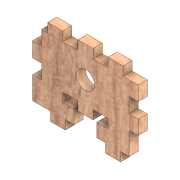
# Autodesk Inventor part: jotstick behuizing zijkant 2.1
Saved by Autodesk Inventor 2020.3 (Build 243373000, 373)
## iProperties
Created: 2020-12-09
Part Number: jotstick behuizing zijkant 2.1
Material: Wood (Birch)
Document SubType Name: Sheet Metal
Designer: Svend
Density: 0.55 g/cm^3
Sheet Metal Rule: Default_mm
Appearance: Birch - Natural Polished
Author: Svend
Autodesk Inventor part; units mm, degrees
ref_plane "YZ Plane" through (0, 0, 0) normal (1, 0, 0) x (0, 1, 0)
ref_plane "XZ Plane" through (0, 0, 0) normal (0, 1, 0) x (-1, 0, 0)
ref_plane "XY Plane" through (0, 0, 0) normal (0, 0, 1) x (1, 0, 0)
ref_plane "Work Plane1" through (20, 0, 0) normal (0, 0, 1) x (1, 0, 0)
sketch "Sketch1" plane through (20, 0, 0) normal (0, 0, 1) x (1, 0, 0)
  line L0 (-20, 0) -> (-10, 0)
  line L1 (-10, 0) -> (-10, 6)
  line L2 (-20, 6) -> (-10, 6)
  line L3 (-20, 0) -> (-20, 6)
  line L4 (0, 0) -> (10, 0)
  line L5 (10, 0) -> (10, 6)
  line L6 (0, 6) -> (10, 6)
  line L7 (0, 0) -> (0, 6)
  line L8 (20, 0) -> (30, 0)
  line L9 (30, 0) -> (30, 6)
  line L10 (20, 6) -> (30, 6)
  line L11 (20, 0) -> (20, 6)
  line L12 (-30, 0) -> (-24, 0)
  line L13 (-24, 0) -> (-24, 6)
  line L14 (-30, 6) -> (-24, 6)
  line L15 (-30, 0) -> (-30, 6)
  line L16 (-30, 0) -> (-20, 0)
  line L17 (-10, 0) -> (0, 0)
  line L18 (10, 0) -> (20, 0)
  line L19 (30, 0) -> (40, 0)
  line L20 (40, 0) -> (-24, 0)
  line L21 (-24, 0) -> (-24, -29)
  line L22 (-24, -29) -> (40, -29)
  line L23 (40, -29) -> (40, 0)
  line L24 (-24, -9.5) -> (-30, -9.5)
  line L25 (-30, -9.5) -> (-30, -19.5)
  line L26 (-30, -19.5) -> (-24, -19.5)
  line L27 (-24, -19.5) -> (-24, -9.5)
  line L28 (40, -19.5) -> (34, -19.5)
  line L29 (34, -19.5) -> (34, -9.5)
  line L30 (34, -9.5) -> (40, -9.5)
  line L31 (40, -9.5) -> (40, -19.5)
  line L32 (-24, -14.5) -> (40, -14.5) construction
  line L33 (-20, -29) -> (-10, -29)
  line L34 (-10, -29) -> (-10, -35)
  line L35 (-20, -35) -> (-10, -35)
  line L36 (-20, -29) -> (-20, -35)
  line L37 (0, -29) -> (10, -29)
  line L38 (10, -29) -> (10, -35)
  line L39 (0, -35) -> (10, -35)
  line L40 (0, -29) -> (0, -35)
  line L41 (20, -29) -> (30, -29)
  line L42 (30, -29) -> (30, -35)
  line L43 (20, -35) -> (30, -35)
  line L44 (20, -29) -> (20, -35)
  line L45 (-10, -29) -> (0, -29)
  line L46 (10, -29) -> (20, -29)
  point P0 (-30, -14.5)
  point P1 (34, -14.5)
  dimension "d0" = 29
  dimension "d1" = 6
  dimension "d2" = 10
  measures "d0" distance of L21.end L20.end
  measures "d1" distance of L26.end L25.end
  measures "d2" distance of L25.end L24.end
extrude "Plate1" add sketch "Sketch1" along normal blind 6 contours L3 L2 L1 L0 | L0 L17 L4 L18 L8 L19 L23 L30 L29 L28 L22 L21 L16 | L7 L6 L5 L4 | L21 L26 L25 L24 | L11 L10 L9 L8 | L22 L34 L35 L36 | L22 L38 L39 L40 | L22 L42 L43 L44
sketch "Sketch2" plane through (20, 0, 6) normal (0, 0, 1) x (1, 0, 0)
  line L0 (-24, -44) -> (-24, -29)
  line L1 (-18.25, -44) -> (-30, -44)
  line L2 (-2.5, -44) -> (-8.25, -44)
  line L3 (-2.5, -35.5) -> (-2.5, -44)
  line L4 (12, -35) -> (-2, -35)
  line L5 (10, -35) -> (0, -35) construction
  line L6 (5, -35) -> (5, 6) construction
  line L7 (0, 6) -> (10, 6) construction
  line L8 (40, -19.5) -> (34, -19.5)
  line L9 (34, -19.5) -> (34, -9.5)
  line L10 (34, -9.5) -> (40, -9.5)
  line L11 (40, 0) -> (40, -9.5)
  line L12 (30, 0) -> (40, 0)
  line L13 (30, 6) -> (30, 0)
  line L14 (20, 6) -> (30, 6)
  line L15 (20, 0) -> (20, 6)
  line L16 (10, 0) -> (20, 0)
  line L17 (10, 6) -> (10, 0)
  line L18 (0, 6) -> (10, 6)
  line L19 (0, 0) -> (0, 6)
  line L20 (-10, 0) -> (0, 0)
  line L21 (-10, 6) -> (-10, 0)
  line L22 (-20, 6) -> (-10, 6)
  line L23 (-20, 0) -> (-20, 6)
  line L24 (-24, 0) -> (-20, 0)
  line L25 (-24, -9.5) -> (-24, 0)
  line L26 (-30, -9.5) -> (-24, -9.5)
  line L27 (-30, -19.5) -> (-30, -9.5)
  line L28 (-24, -19.5) -> (-30, -19.5)
  line L29 (-24, -29) -> (-24, -19.5)
  line L30 (-20, -29) -> (-24, -29)
  line L31 (-20, -35) -> (-20, -29)
  line L32 (-10, -35) -> (-20, -35)
  line L33 (-10, -29) -> (-10, -35)
  line L34 (0, -29) -> (-10, -29)
  line L35 (0, -35) -> (0, -29)
  line L36 (10, -35) -> (0, -35)
  line L37 (10, -29) -> (10, -35)
  line L38 (20, -29) -> (10, -29)
  line L39 (20, -35) -> (20, -29)
  line L40 (30, -35) -> (20, -35)
  line L41 (30, -29) -> (30, -35)
  line L42 (40, -29) -> (30, -29)
  line L43 (40, -19.5) -> (40, -29)
  line L44 (-2.5, -44) -> (-2.5, -35)
  line L45 (-2.5, -35) -> (0, -35)
  line L46 (-8.25, -50) -> (-18.25, -50)
  line L47 (-18.25, -50) -> (-18.25, -44)
  line L48 (34, -44) -> (34, -29)
  line L49 (12.5, -44) -> (18.25, -44)
  line L50 (12.5, -35.5) -> (12.5, -44)
  line L51 (30, -29) -> (34, -29)
  line L52 (30, -35) -> (30, -29)
  line L53 (20, -35) -> (30, -35)
  line L54 (20, -29) -> (20, -35)
  line L55 (10, -29) -> (20, -29)
  line L56 (10, -35) -> (10, -29)
  line L57 (12.5, -44) -> (12.5, -35)
  line L58 (12.5, -35) -> (10, -35)
  line L59 (18.25, -50) -> (28.25, -50)
  line L60 (28.25, -50) -> (28.25, -44)
  line L61 (28.25, -44) -> (34, -44)
  line L62 (-24, -29) -> (-20, -29)
  line L63 (-20, -35) -> (-20, -29)
  line L64 (-20, -35) -> (-20, -29)
  line L65 (-20, -35) -> (-10, -35)
  line L66 (-10, -35) -> (-10, -29)
  line L67 (0, -29) -> (-10, -29)
  line L68 (0, -29) -> (0, -35)
  line L69 (-8.25, -44) -> (-8.25, -50)
  line L70 (18.25, -50) -> (18.25, -44)
  line L71 (34, -44) -> (34, -29)
  line L72 (28.25, -44) -> (40, -44)
  line L73 (12.5, -44) -> (18.25, -44)
  line L74 (12.5, -35.5) -> (12.5, -44)
  line L75 (30, -29) -> (34, -29)
  line L76 (30, -35) -> (30, -29)
  line L77 (20, -35) -> (30, -35)
  line L78 (20, -29) -> (20, -35)
  line L79 (10, -29) -> (20, -29)
  line L80 (10, -35) -> (10, -29)
  line L81 (12.5, -44) -> (12.5, -35)
  line L82 (12.5, -35) -> (10, -35)
  line L83 (18.25, -50) -> (28.25, -50)
  line L84 (28.25, -50) -> (28.25, -44)
  line L85 (34, -29) -> (30, -29)
  line L86 (30, -35) -> (30, -29)
  line L87 (30, -35) -> (30, -29)
  line L88 (30, -35) -> (20, -35)
  line L89 (20, -35) -> (20, -29)
  line L90 (10, -29) -> (20, -29)
  line L91 (10, -29) -> (10, -35)
  line L92 (18.25, -44) -> (18.25, -50)
  line L93 (-24, -44) -> (-30, -44)
  line L94 (-30, -44) -> (-30, -29)
  line L95 (-30, -29) -> (-24, -29)
  line L96 (-24, -29) -> (-24, -44)
  line L97 (-10, -29) -> (0, -29)
  line L98 (0, -29) -> (0, -35)
  line L99 (0, -35) -> (-10, -35)
  line L100 (-10, -35) -> (-10, -29)
  line L101 (20, -29) -> (10, -29)
  line L102 (10, -29) -> (20, -29)
  line L103 (20, -29) -> (20, -35)
  line L104 (20, -35) -> (10, -35)
  line L105 (10, -35) -> (10, -29)
  line L106 (30, -29) -> (34, -29)
  line L107 (34, -29) -> (34, -35)
  line L108 (34, -35) -> (30, -35)
  line L109 (30, -35) -> (30, -29)
  line L110 (-20, -29) -> (-24, -29)
  line L111 (-24, -29) -> (-24, -35)
  line L112 (-24, -35) -> (-20, -35)
  line L113 (-20, -35) -> (-20, -29)
  line L114 (30, -35) -> (20, -35)
  point P0 (-2.5, -49.5)
  point P1 (12.5, -49.5)
  point P2 (12.5, -49.5)
  dimension "d4" = 10
  dimension "d6" = 6
  dimension "d12" = 6
  dimension "d13" = 15
  measures "d4" distance of L46.start L46.end
  measures "d6" distance of L2.end L46.start
  measures "d12" distance of L94.end L95.end
  measures "d13" distance of L93.end L94.end
sheet face with bend "Face2" sketch "Sketch2" thickness 6 toward (0, 0, -1) bend radius 6 contours L1 L94 L95 L0 | L0 L112 L32 L99 L44 L3 L2 L69 L46 L47 L1 | L0 L30 L31 L112 | L104 L40 L108 L48 L61 L60 L59 L70 L49 L50 L57 | L41 L42 L48 L108
bend "Bend1"
sketch "Sketch3" plane through (20, 0, 6) normal (0, 0, 1) x (1, 0, 0)
  line L0 (40, -19.5) -> (34, -19.5) projected
  line L1 (34, -19.5) -> (34, -9.5) projected
  line L2 (34, -9.5) -> (40, -9.5) projected
  line L3 (40, 0) -> (40, -9.5) projected
  line L4 (30, 0) -> (40, 0) projected
  line L5 (30, 6) -> (30, 0) projected
  line L6 (20, 6) -> (30, 6) projected
  line L7 (20, 0) -> (20, 6) projected
  line L8 (10, 0) -> (20, 0) projected
  line L9 (10, 6) -> (10, 0) projected
  line L10 (0, 6) -> (10, 6) projected
  line L11 (0, 0) -> (0, 6) projected
  line L12 (-10, 0) -> (0, 0) projected
  line L13 (-10, 6) -> (-10, 0) projected
  line L14 (-20, 6) -> (-10, 6) projected
  line L15 (-20, 0) -> (-20, 6) projected
  line L16 (-24, 0) -> (-20, 0) projected
  line L17 (-24, -9.5) -> (-24, 0) projected
  line L18 (-30, -9.5) -> (-24, -9.5) projected
  line L19 (-30, -19.5) -> (-30, -9.5) projected
  line L20 (-24, -19.5) -> (-30, -19.5) projected
  line L21 (-24, -29) -> (-24, -19.5) projected
  line L22 (-24, -29) -> (-30, -29) projected
  line L23 (-30, -29) -> (-30, -44) projected
  line L24 (-30, -44) -> (-18.25, -44) projected
  line L25 (-18.25, -44) -> (-18.25, -50) projected
  line L26 (-18.25, -50) -> (-8.25, -50) projected
  line L27 (-8.25, -50) -> (-8.25, -44) projected
  line L28 (-8.25, -44) -> (-2.5, -44) projected
  line L29 (-2.5, -44) -> (-2.5, -35) projected
  line L30 (-2.5, -35) -> (-10, -35) projected
  line L31 (-10, -29) -> (-10, -35) projected
  line L32 (0, -29) -> (-10, -29) projected
  line L33 (0, -35) -> (0, -29) projected
  line L34 (10, -35) -> (0, -35) projected
  line L35 (10, -29) -> (10, -35) projected
  line L36 (20, -29) -> (10, -29) projected
  line L37 (20, -35) -> (20, -29) projected
  line L38 (20, -35) -> (12.5, -35) projected
  line L39 (12.5, -35) -> (12.5, -44) projected
  line L40 (12.5, -44) -> (18.25, -44) projected
  line L41 (18.25, -44) -> (18.25, -50) projected
  line L42 (18.25, -50) -> (28.25, -50) projected
  line L43 (28.25, -50) -> (28.25, -44) projected
  line L44 (28.25, -44) -> (34, -44) projected
  line L45 (34, -44) -> (34, -29) projected
  line L46 (40, -29) -> (34, -29) projected
  line L47 (40, -19.5) -> (40, -29) projected
  circle A0 centre (5, -14.5) radius 6
  point P0 (5, 6)
  point P1 (34, -14.5)
  dimension "d14" = 12
  constraints: 2 midpoint, 1 centre point, 1 horizontal alignment, 1 vertical alignment
  measures "d14" diameter of A0
extrude "Cut1" cut sketch "Sketch3" against normal blind 6 contours A0
equation "\"d12\" = d6"
equation "\"d15\" = Thickness"
equation "\"d3\" = Thickness"
equation "\"d7\" = BendRadius"
equation "\"d8\" = BendReliefWidth"
equation "\"d10\" = MinimumRemnant"
equation "\"d9\" = BendReliefDepth"
equation "\"d11\" = TransitionRadius"
equation "\"BendRadius\" = Thickness"
equation "\"BendReliefWidth\" = Thickness"
equation "\"BendReliefDepth\" = 0.5 * Thickness"
equation "\"CornerReliefSize\" = 4 * Thickness"
equation "\"MinimumRemnant\" = 2 * Thickness"
equation "\"TransitionRadius\" = BendRadius"
equation "\"JacobiRadiusSize\" = BendRadius"
equation "\"GapSize\" = Thickness"
equation "\"Thickness\" = 6"
body "Solid1"
